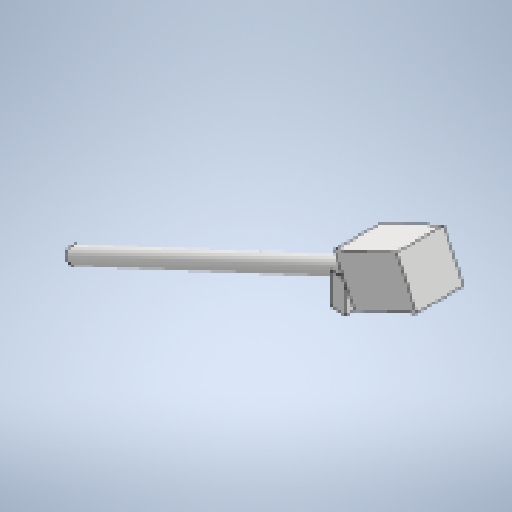
# Autodesk Inventor part: NDM-VOS dummy5
Saved by Autodesk Inventor 2025 (Build 290162010, 162A)
## iProperties
Created: 2024-10-01
Part Number: NDM-VOS dummy5
Material: Generic
Document SubType Name: Modeling
Designer: pokla
Density: 1 g/cm^3
Appearance: Default
Author: pokla
Autodesk Inventor part; units mm, degrees
ref_plane "YZ Plane" through (0, 0, 0) normal (1, 0, 0) x (0, 1, 0)
ref_plane "XZ Plane" through (0, 0, 0) normal (0, 1, 0) x (-1, 0, 0)
ref_plane "XY Plane" through (0, 0, 0) normal (0, 0, 1) x (1, 0, 0)
sketch "Sketch2" plane through (0, 0, 0) normal (0, 1, 0) x (-1, 0, 0)
  line L0 (1359.4617, 1616.0726) -> (-453.1539, 2461.3091)
  line L1 (1359.4617, 1616.0726) -> (-640.5383, 1616.0726) construction
  line L2 (0, 0) -> (0, 2250)
  line L3 (-389.7612, 2597.2553) -> (-842.915, 2808.5644)
  line L4 (-842.915, 2808.5644) -> (-969.7005, 2536.6721)
  line L5 (-969.7005, 2536.6721) -> (-516.5466, 2325.363)
  line L6 (-516.5466, 2325.363) -> (-389.7612, 2597.2553)
  line L7 (-444.1396, 2622.6124) -> (-570.9251, 2350.7201)
  line L8 (-475.836, 2554.6393) -> (-421.4575, 2529.2822)
  line L9 (-539.2287, 2418.6931) -> (-484.8503, 2393.336)
  line L10 (-317.2077, 2397.9164) -> (-417.2077, 2397.9164)
  line L11 (-417.2077, 2397.9164) -> (-417.2077, 2197.9164)
  line L12 (-417.2077, 2197.9164) -> (-317.2077, 2197.9164)
  line L13 (-317.2077, 2197.9164) -> (-317.2077, 2397.9164)
  line L14 (-317.2077, 2397.9164) -> (-417.2077, 2197.9164) construction
  line L15 (-417.2077, 2397.9164) -> (-317.2077, 2197.9164) construction
  point P0 (-367.2077, 2297.9164)
  dimension "d3" = 25
  dimension "d4" = 2000
  dimension "d10" = 2250
  dimension "d11" = 500
  dimension "d12" = 500
  dimension "d13" = 300
  dimension "d14" = 150
  dimension "d15" = 60
  dimension "d16" = 100
  dimension "d17" = 200
  dimension "d18" = 150
  constraints: 32 end point, 8 point on line, 5 parallel, 5 perpendicular, 3 midpoint, 2 horizontal, 1 equal length, 1 vertical, 1 other
  measures "d3" angle of L1 L0
  measures "d4" distance of L0.end L0.start
  measures "d10" distance of L2.start L2.end
  measures "d11" distance of L0.end L2.end
  measures "d12" distance of L3.start L3.end
  measures "d13" distance of L5.end L3.start
  measures "d14" distance between parallel lines of L9 L8
  measures "d15" distance of L9.start L9.end
  measures "d16" distance of L11.end L12.end
  measures "d17" distance of L12.end L10.start
  measures "d18" distance of L10.start L0.end
ref_plane "Work Plane1" through (-1359.4617, 0, 1616.0726) normal (0.9063078, 0, 0.4226183) x (0, 1, 0)
sketch "Sketch3" plane through (-1359.4617, 0, 1616.0726) normal (0.9063078, 0, 0.4226183) x (0, 1, 0)
  circle A0 centre (0, 0) radius 50
  circle A1 centre (0, 0) radius 47
  point P0 (0, -2039.1925)
  dimension "d6" = 100
  dimension "d7" = 3
  constraints: 2 centre point, 1 coincident
  measures "d6" diameter of A0
  measures "d7" radial gap between concentric circles of A0 A1
sweep "Sweep1" add profiles "Sketch3" path "Sketch2" path curves L0
extrude "Extrusion2" add sketch "Sketch2" along normal mid plane 100 contours L6 L9 L7 L8 | L13 L12 L11 L10
extrude "Extrusion3" add sketch "Sketch2" along normal mid plane 300 contours L7 L5 L4 L3
equation "\"d16\" = d6"
equation "\"d19\" = d6"
body "Solid2"
